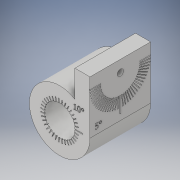
# Autodesk Inventor part: cam_holder_end_part
Saved by Autodesk Inventor 2019 (Build 230136000, 136)
## iProperties
Created: 2024-08-06
Part Number: cam_holder_end_part
Material: Generisch
Document SubType Name: Modeling
Designer: nic
Density: 1 g/cm^3
Appearance: Vorgabe
Author: nic
Autodesk Inventor part; units mm, degrees
ref_plane "YZ Plane" through (0, 0, 0) normal (1, 0, 0) x (0, 1, 0)
ref_plane "XY Plane" through (0, 0, 0) normal (0, 0, 1) x (1, 0, 0)
sketch "Skizze1" plane through (0, 0, 0) normal (0, 0, 1) x (1, 0, 0)
  circle A0 centre (0, 0) radius 10.05
  circle A1 centre (0, 0) radius 20
  line L0 (20, 0) -> (10.05, 0)
  line L1 (10.05, 0) -> (10.05, 35)
  line L2 (10.05, 35) -> (20, 35)
  line L3 (20, 35) -> (20, 0)
  dimension "d1" = 40
  dimension "d0" = 20.1
  dimension "d2" = 35
  constraints: 8 end point, 2 coincident, 2 parallel, 1 centre point, 1 horizontal, 1 horizontal alignment, 1 perpendicular, 2 other
  measures "d0" diameter of A0
  measures "d2" distance of L0.end L1.end
extrude "Extrusion1" add sketch "Skizze1" along normal blind 40
sketch "Skizze2" plane through (0, 0, 40) normal (0, 0, 1) x (1, 0, 0)
  line L0 (7.55, 0.25) -> (12.55, 0.25)
  line L1 (12.55, 0.25) -> (12.55, -0.25)
  line L2 (12.55, -0.25) -> (7.55, -0.25)
  line L3 (7.55, -0.25) -> (7.55, 0.25)
  circle A0 centre (0, 0) radius 10.05 projected
  line L4 (7.55, 0.25) -> (12.55, -0.25) construction
  line L5 (12.55, 0.25) -> (7.55, -0.25) construction
  line L6 (7.384, 1.5941) -> (12.3037, 2.4869)
  line L7 (12.3037, 2.4869) -> (12.393, 1.9949)
  line L8 (12.393, 1.9949) -> (7.4733, 1.1021)
  line L9 (7.4733, 1.1021) -> (7.384, 1.5941)
  line L10 (7.384, 1.5941) -> (12.393, 1.9949) construction
  line L11 (12.3037, 2.4869) -> (7.4733, 1.1021) construction
  line L12 (6.9807, 2.8869) -> (11.6619, 4.6438)
  line L13 (11.6619, 4.6438) -> (11.8376, 4.1757)
  line L14 (11.8376, 4.1757) -> (7.1564, 2.4188)
  line L15 (7.1564, 2.4188) -> (6.9807, 2.8869)
  line L16 (6.9807, 2.8869) -> (11.8376, 4.1757) construction
  line L17 (11.6619, 4.6438) -> (7.1564, 2.4188) construction
  line L18 (6.3531, 4.087) -> (10.6453, 6.6515)
  line L19 (10.6453, 6.6515) -> (10.9018, 6.2223)
  line L20 (10.9018, 6.2223) -> (6.6095, 3.6578)
  line L21 (6.6095, 3.6578) -> (6.3531, 4.087)
  line L22 (6.3531, 4.087) -> (10.9018, 6.2223) construction
  line L23 (10.6453, 6.6515) -> (6.6095, 3.6578) construction
  line L24 (5.5212, 5.1557) -> (9.2866, 8.4454)
  line L25 (9.2866, 8.4454) -> (9.6155, 8.0689)
  line L26 (9.6155, 8.0689) -> (5.8502, 4.7792)
  line L27 (5.8502, 4.7792) -> (5.5212, 5.1557)
  line L28 (5.5212, 5.1557) -> (9.6155, 8.0689) construction
  line L29 (9.2866, 8.4454) -> (5.8502, 4.7792) construction
  line L30 (4.5119, 6.0587) -> (7.6293, 9.9679)
  line L31 (7.6293, 9.9679) -> (8.0203, 9.6561)
  line L32 (8.0203, 9.6561) -> (4.9028, 5.747)
  line L33 (4.9028, 5.747) -> (4.5119, 6.0587)
  line L34 (4.5119, 6.0587) -> (8.0203, 9.6561) construction
  line L35 (7.6293, 9.9679) -> (4.9028, 5.747) construction
  line L36 (3.3576, 6.767) -> (5.7269, 11.1699)
  line L37 (5.7269, 11.1699) -> (6.1672, 10.933)
  line L38 (6.1672, 10.933) -> (3.7979, 6.53)
  line L39 (3.7979, 6.53) -> (3.3576, 6.767)
  line L40 (3.3576, 6.767) -> (6.1672, 10.933) construction
  line L41 (5.7269, 11.1699) -> (3.7979, 6.53) construction
  line L42 (2.0953, 7.2577) -> (3.6404, 12.013)
  line L43 (3.6404, 12.013) -> (4.1159, 11.8585)
  line L44 (4.1159, 11.8585) -> (2.5708, 7.1032)
  line L45 (2.5708, 7.1032) -> (2.0953, 7.2577)
  line L46 (2.0953, 7.2577) -> (4.1159, 11.8585) construction
  line L47 (3.6404, 12.013) -> (2.5708, 7.1032) construction
  line L48 (0.7657, 7.5152) -> (1.4369, 12.47)
  line L49 (1.4369, 12.47) -> (1.9324, 12.4029)
  line L50 (1.9324, 12.4029) -> (1.2612, 7.4481)
  line L51 (1.2612, 7.4481) -> (0.7657, 7.5152)
  line L52 (0.7657, 7.5152) -> (1.9324, 12.4029) construction
  line L53 (1.4369, 12.47) -> (1.2612, 7.4481) construction
  line L54 (-0.5885, 7.5312) -> (-0.8128, 12.5261)
  line L55 (-0.8128, 12.5261) -> (-0.3133, 12.5486)
  line L56 (-0.3133, 12.5486) -> (-0.089, 7.5536)
  line L57 (-0.089, 7.5536) -> (-0.5885, 7.5312)
  line L58 (-0.5885, 7.5312) -> (-0.3133, 12.5486) construction
  line L59 (-0.8128, 12.5261) -> (-0.089, 7.5536) construction
  line L60 (-1.9238, 7.3051) -> (-3.0364, 12.1797)
  line L61 (-3.0364, 12.1797) -> (-2.5489, 12.291)
  line L62 (-2.5489, 12.291) -> (-1.4363, 7.4163)
  line L63 (-1.4363, 7.4163) -> (-1.9238, 7.3051)
  line L64 (-1.9238, 7.3051) -> (-2.5489, 12.291) construction
  line L65 (-3.0364, 12.1797) -> (-1.4363, 7.4163) construction
  line L66 (-3.1972, 6.8442) -> (-5.1623, 11.4418)
  line L67 (-5.1623, 11.4418) -> (-4.7026, 11.6383)
  line L68 (-4.7026, 11.6383) -> (-2.7375, 7.0407)
  line L69 (-2.7375, 7.0407) -> (-3.1972, 6.8442)
  line L70 (-3.1972, 6.8442) -> (-4.7026, 11.6383) construction
  line L71 (-5.1623, 11.4418) -> (-2.7375, 7.0407) construction
  line L72 (-4.3679, 6.1633) -> (-7.1224, 10.3362)
  line L73 (-7.1224, 10.3362) -> (-6.7051, 10.6116)
  line L74 (-6.7051, 10.6116) -> (-3.9506, 6.4388)
  line L75 (-3.9506, 6.4388) -> (-4.3679, 6.1633)
  line L76 (-4.3679, 6.1633) -> (-6.7051, 10.6116) construction
  line L77 (-7.1224, 10.3362) -> (-3.9506, 6.4388) construction
  line L78 (-5.3982, 5.2843) -> (-8.8535, 8.8983)
  line L79 (-8.8535, 8.8983) -> (-8.4921, 9.2438)
  line L80 (-8.4921, 9.2438) -> (-5.0368, 5.6299)
  line L81 (-5.0368, 5.6299) -> (-5.3982, 5.2843)
  line L82 (-5.3982, 5.2843) -> (-8.4921, 9.2438) construction
  line L83 (-8.8535, 8.8983) -> (-5.0368, 5.6299) construction
  line L84 (-6.255, 4.2355) -> (-10.3001, 7.1745)
  line L85 (-10.3001, 7.1745) -> (-10.0062, 7.579)
  line L86 (-10.0062, 7.579) -> (-5.9611, 4.64)
  line L87 (-5.9611, 4.64) -> (-6.255, 4.2355)
  line L88 (-6.255, 4.2355) -> (-10.0062, 7.579) construction
  line L89 (-10.3001, 7.1745) -> (-5.9611, 4.64) construction
  line L90 (-6.9108, 3.0506) -> (-11.4156, 5.22)
  line L91 (-11.4156, 5.22) -> (-11.1987, 5.6705)
  line L92 (-11.1987, 5.6705) -> (-6.6938, 3.5011)
  line L93 (-6.6938, 3.5011) -> (-6.9108, 3.0506)
  line L94 (-6.9108, 3.0506) -> (-11.1987, 5.6705) construction
  line L95 (-11.4156, 5.22) -> (-6.6938, 3.5011) construction
  line L96 (-7.3444, 1.7676) -> (-12.1642, 3.0978)
  line L97 (-12.1642, 3.0978) -> (-12.0312, 3.5798)
  line L98 (-12.0312, 3.5798) -> (-7.2114, 2.2496)
  line L99 (-7.2114, 2.2496) -> (-7.3444, 1.7676)
  line L100 (-7.3444, 1.7676) -> (-12.0312, 3.5798) construction
  line L101 (-12.1642, 3.0978) -> (-7.2114, 2.2496) construction
  line L102 (-7.542, 0.4278) -> (-12.5219, 0.876)
  line L103 (-12.5219, 0.876) -> (-12.4771, 1.374)
  line L104 (-12.4771, 1.374) -> (-7.4972, 0.9258)
  line L105 (-7.4972, 0.9258) -> (-7.542, 0.4278)
  line L106 (-7.542, 0.4278) -> (-12.4771, 1.374) construction
  line L107 (-12.5219, 0.876) -> (-7.4972, 0.9258) construction
  line L108 (-7.4972, -0.9258) -> (-12.4771, -1.374)
  line L109 (-12.4771, -1.374) -> (-12.5219, -0.876)
  line L110 (-12.5219, -0.876) -> (-7.542, -0.4278)
  line L111 (-7.542, -0.4278) -> (-7.4972, -0.9258)
  line L112 (-7.4972, -0.9258) -> (-12.5219, -0.876) construction
  line L113 (-12.4771, -1.374) -> (-7.542, -0.4278) construction
  line L114 (-7.2114, -2.2496) -> (-12.0312, -3.5798)
  line L115 (-12.0312, -3.5798) -> (-12.1642, -3.0978)
  line L116 (-12.1642, -3.0978) -> (-7.3444, -1.7676)
  line L117 (-7.3444, -1.7676) -> (-7.2114, -2.2496)
  line L118 (-7.2114, -2.2496) -> (-12.1642, -3.0978) construction
  line L119 (-12.0312, -3.5798) -> (-7.3444, -1.7676) construction
  line L120 (-6.6938, -3.5011) -> (-11.1987, -5.6705)
  line L121 (-11.1987, -5.6705) -> (-11.4156, -5.22)
  line L122 (-11.4156, -5.22) -> (-6.9108, -3.0506)
  line L123 (-6.9108, -3.0506) -> (-6.6938, -3.5011)
  line L124 (-6.6938, -3.5011) -> (-11.4156, -5.22) construction
  line L125 (-11.1987, -5.6705) -> (-6.9108, -3.0506) construction
  line L126 (-5.9611, -4.64) -> (-10.0062, -7.579)
  line L127 (-10.0062, -7.579) -> (-10.3001, -7.1745)
  line L128 (-10.3001, -7.1745) -> (-6.255, -4.2355)
  line L129 (-6.255, -4.2355) -> (-5.9611, -4.64)
  line L130 (-5.9611, -4.64) -> (-10.3001, -7.1745) construction
  line L131 (-10.0062, -7.579) -> (-6.255, -4.2355) construction
  line L132 (-5.0368, -5.6299) -> (-8.4921, -9.2438)
  line L133 (-8.4921, -9.2438) -> (-8.8535, -8.8983)
  line L134 (-8.8535, -8.8983) -> (-5.3982, -5.2843)
  line L135 (-5.3982, -5.2843) -> (-5.0368, -5.6299)
  line L136 (-5.0368, -5.6299) -> (-8.8535, -8.8983) construction
  line L137 (-8.4921, -9.2438) -> (-5.3982, -5.2843) construction
  line L138 (-3.9506, -6.4388) -> (-6.7051, -10.6116)
  line L139 (-6.7051, -10.6116) -> (-7.1224, -10.3362)
  line L140 (-7.1224, -10.3362) -> (-4.3679, -6.1633)
  line L141 (-4.3679, -6.1633) -> (-3.9506, -6.4388)
  line L142 (-3.9506, -6.4388) -> (-7.1224, -10.3362) construction
  line L143 (-6.7051, -10.6116) -> (-4.3679, -6.1633) construction
  line L144 (-2.7375, -7.0407) -> (-4.7026, -11.6383)
  line L145 (-4.7026, -11.6383) -> (-5.1623, -11.4418)
  line L146 (-5.1623, -11.4418) -> (-3.1972, -6.8442)
  line L147 (-3.1972, -6.8442) -> (-2.7375, -7.0407)
  line L148 (-2.7375, -7.0407) -> (-5.1623, -11.4418) construction
  line L149 (-4.7026, -11.6383) -> (-3.1972, -6.8442) construction
  line L150 (-1.4363, -7.4163) -> (-2.5489, -12.291)
  line L151 (-2.5489, -12.291) -> (-3.0364, -12.1797)
  line L152 (-3.0364, -12.1797) -> (-1.9238, -7.3051)
  line L153 (-1.9238, -7.3051) -> (-1.4363, -7.4163)
  line L154 (-1.4363, -7.4163) -> (-3.0364, -12.1797) construction
  line L155 (-2.5489, -12.291) -> (-1.9238, -7.3051) construction
  line L156 (-0.089, -7.5536) -> (-0.3133, -12.5486)
  line L157 (-0.3133, -12.5486) -> (-0.8128, -12.5261)
  line L158 (-0.8128, -12.5261) -> (-0.5885, -7.5312)
  line L159 (-0.5885, -7.5312) -> (-0.089, -7.5536)
  line L160 (-0.089, -7.5536) -> (-0.8128, -12.5261) construction
  line L161 (-0.3133, -12.5486) -> (-0.5885, -7.5312) construction
  line L162 (1.2612, -7.4481) -> (1.9324, -12.4029)
  line L163 (1.9324, -12.4029) -> (1.4369, -12.47)
  line L164 (1.4369, -12.47) -> (0.7657, -7.5152)
  line L165 (0.7657, -7.5152) -> (1.2612, -7.4481)
  line L166 (1.2612, -7.4481) -> (1.4369, -12.47) construction
  line L167 (1.9324, -12.4029) -> (0.7657, -7.5152) construction
  line L168 (2.5708, -7.1032) -> (4.1159, -11.8585)
  line L169 (4.1159, -11.8585) -> (3.6404, -12.013)
  line L170 (3.6404, -12.013) -> (2.0953, -7.2577)
  line L171 (2.0953, -7.2577) -> (2.5708, -7.1032)
  line L172 (2.5708, -7.1032) -> (3.6404, -12.013) construction
  line L173 (4.1159, -11.8585) -> (2.0953, -7.2577) construction
  line L174 (3.7979, -6.53) -> (6.1672, -10.933)
  line L175 (6.1672, -10.933) -> (5.7269, -11.1699)
  line L176 (5.7269, -11.1699) -> (3.3576, -6.767)
  line L177 (3.3576, -6.767) -> (3.7979, -6.53)
  line L178 (3.7979, -6.53) -> (5.7269, -11.1699) construction
  line L179 (6.1672, -10.933) -> (3.3576, -6.767) construction
  line L180 (4.9028, -5.747) -> (8.0203, -9.6561)
  line L181 (8.0203, -9.6561) -> (7.6293, -9.9679)
  line L182 (7.6293, -9.9679) -> (4.5119, -6.0587)
  line L183 (4.5119, -6.0587) -> (4.9028, -5.747)
  line L184 (4.9028, -5.747) -> (7.6293, -9.9679) construction
  line L185 (8.0203, -9.6561) -> (4.5119, -6.0587) construction
  line L186 (5.8502, -4.7792) -> (9.6155, -8.0689)
  line L187 (9.6155, -8.0689) -> (9.2866, -8.4454)
  line L188 (9.2866, -8.4454) -> (5.5212, -5.1557)
  line L189 (5.5212, -5.1557) -> (5.8502, -4.7792)
  line L190 (5.8502, -4.7792) -> (9.2866, -8.4454) construction
  line L191 (9.6155, -8.0689) -> (5.5212, -5.1557) construction
  line L192 (6.6095, -3.6578) -> (10.9018, -6.2223)
  line L193 (10.9018, -6.2223) -> (10.6453, -6.6515)
  line L194 (10.6453, -6.6515) -> (6.3531, -4.087)
  line L195 (6.3531, -4.087) -> (6.6095, -3.6578)
  line L196 (6.6095, -3.6578) -> (10.6453, -6.6515) construction
  line L197 (10.9018, -6.2223) -> (6.3531, -4.087) construction
  line L198 (7.1564, -2.4188) -> (11.8376, -4.1757)
  line L199 (11.8376, -4.1757) -> (11.6619, -4.6438)
  line L200 (11.6619, -4.6438) -> (6.9807, -2.8869)
  line L201 (6.9807, -2.8869) -> (7.1564, -2.4188)
  line L202 (7.1564, -2.4188) -> (11.6619, -4.6438) construction
  line L203 (11.8376, -4.1757) -> (6.9807, -2.8869) construction
  line L204 (7.4733, -1.1021) -> (12.393, -1.9949)
  line L205 (12.393, -1.9949) -> (12.3037, -2.4869)
  line L206 (12.3037, -2.4869) -> (7.384, -1.5941)
  line L207 (7.384, -1.5941) -> (7.4733, -1.1021)
  line L208 (7.4733, -1.1021) -> (12.3037, -2.4869) construction
  line L209 (12.393, -1.9949) -> (7.384, -1.5941) construction
  line L210 (4.9213, 0.25) -> (15.1787, 0.25)
  line L211 (15.1787, 0.25) -> (15.1787, -0.25)
  line L212 (15.1787, -0.25) -> (4.9213, -0.25)
  line L213 (4.9213, -0.25) -> (4.9213, 0.25)
  line L214 (4.9213, 0.25) -> (15.1787, -0.25) construction
  line L215 (15.1787, 0.25) -> (4.9213, -0.25) construction
  point P0 (10.05, 0)
  point P1 (9.8885, 1.7945)
  point P2 (9.4092, 3.5313)
  point P3 (8.6274, 5.1546)
  point P4 (7.5684, 6.6123)
  point P5 (6.2661, 7.8574)
  point P6 (4.7624, 8.85)
  point P7 (3.1056, 9.5581)
  point P8 (1.349, 9.959)
  point P9 (-0.4509, 10.0399)
  point P10 (-2.2363, 9.798)
  point P11 (-3.9499, 9.2413)
  point P12 (-5.5365, 8.3875)
  point P13 (-6.9452, 7.2641)
  point P14 (-8.1306, 5.9072)
  point P15 (-9.0547, 4.3605)
  point P16 (-9.6878, 2.6737)
  point P17 (-10.0095, 0.9009)
  point P18 (-10.0095, -0.9009)
  point P19 (-9.6878, -2.6737)
  point P20 (-9.0547, -4.3605)
  point P21 (-8.1306, -5.9072)
  point P22 (-6.9452, -7.2641)
  point P23 (-5.5365, -8.3875)
  point P24 (-3.9499, -9.2413)
  point P25 (-2.2363, -9.798)
  point P26 (-0.4509, -10.0399)
  point P27 (1.349, -9.959)
  point P28 (3.1056, -9.5581)
  point P29 (4.7624, -8.85)
  point P30 (6.2661, -7.8574)
  point P31 (7.5684, -6.6123)
  point P32 (8.6274, -5.1546)
  point P33 (9.4092, -3.5313)
  point P34 (9.8885, -1.7945)
  dimension "d5" = 5
  dimension "d6" = 0.5
  dimension "d9" = 360
  constraints: 432 end point, 72 midpoint, 4 parallel, 2 horizontal, 2 perpendicular, 1 horizontal alignment, 387 other
  measures "d5" distance of L1.end L2.end
  measures "d6" distance of L0.end L1.end
extrude "Extrusion2" cut sketch "Skizze2" against normal blind 0.5 contours L0 A0 L2 L3 | L3 L212 L213 L210 | L0 L1 L2 A0 | L210 L211 L212 L1 | L8 L9 L6 A0 | A0 L6 L7 L8 | L204 L205 L206 A0 | A0 L206 L207 L204 | L14 L15 L12 A0 | A0 L12 L13 L14 | L198 L199 L200 A0 | A0 L200 L201 L198 | L20 L21 L18 A0 | A0 L18 L19 L20 | L192 L193 L194 A0 | A0 L194 L195 L192 | L26 L27 L24 A0 | A0 L24 L25 L26 | L186 L187 L188 A0 | A0 L188 L189 L186 | L32 L33 L30 A0 | A0 L30 L31 L32 | L180 L181 L182 A0 | A0 L182 L183 L180 | L38 L39 L36 A0 | A0 L36 L37 L38 | L174 L175 L176 A0 | A0 L176 L177 L174 | L44 L45 L42 A0 | A0 L42 L43 L44 | L168 L169 L170 A0 | A0 L170 L171 L168 | L50 L51 L48 A0 | A0 L48 L49 L50 | L162 L163 L164 A0 | A0 L164 L165 L162 | L56 L57 L54 A0 | A0 L54 L55 L56 | L156 L157 L158 A0 | A0 L158 L159 L156 | L62 L63 L60 A0 | A0 L60 L61 L62 | L150 L151 L152 A0 | A0 L152 L153 L150 | L68 L69 L66 A0 | A0 L66 L67 L68 | L144 L145 L146 A0 | A0 L146 L147 L144 | L74 L75 L72 A0 | A0 L72 L73 L74 | L138 L139 L140 A0 | A0 L140 L141 L138 | L80 L81 L78 A0 | A0 L78 L79 L80 | L132 L133 L134 A0 | A0 L134 L135 L132 | L86 L87 L84 A0 | A0 L84 L85 L86 | L126 L127 L128 A0 | A0 L128 L129 L126 | L92 L93 L90 A0 | A0 L90 L91 L92 | L120 L121 L122 A0 | A0 L122 L123 L120 | L98 L99 L96 A0 | A0 L96 L97 L98 | L114 L115 L116 A0 | A0 L116 L117 L114 | L104 L105 L102 A0 | A0 L102 L103 L104 | L108 L109 L110 A0 | A0 L110 L111 L108
sketch "Skizze3" plane through (10.05, 17.2915, 0) normal (-1, 0, 0) x (0, 0, 1)
  line L0 (0, 0) -> (40, 0) construction
  line L1 (40, 17.7085) -> (40, 0) construction
  line L2 (0, 17.7085) -> (40, 17.7085) construction
  line L3 (0, 0) -> (0, 17.7085) construction
  line L4 (0, 17.7085) -> (40, 17.7085) projected
  line L5 (20, 17.7085) -> (20, 7.753)
  line L6 (40, 17.7085) -> (40, 0) projected
  line L7 (40, 10.1178) -> (0, 10.1178)
  point P0 (0, -17.2915)
  point P1 (20, 10.1178)
  constraints: 4 end point, 2 midpoint, 2 point on line, 1 perpendicular, 1 vertical
hole "Bohrung1" at (10.05, 27.4094, 20) direction (1, 0, 0) diameter 4.1 depth 20 tip angle 118 counterbore diameter 8 counterbore depth 3 clearance for "Zylinderschraube mit Schlitz DIN 84" size "M4" standard "DIN"
ref_plane "Arbeitsebene1" through (0, -20, 0) normal (0, 1, 0) x (-1, 0, 0)
sketch "Skizze4" plane through (0, -20, 0) normal (0, 1, 0) x (-1, 0, 0)
  line L0 (-10.05, 0) -> (-10.05, 40) construction
  line L1 (-20, 0) -> (-10.05, 0) construction
  line L2 (-20, 0) -> (-20, 40) construction
  line L3 (-10.05, 40) -> (-20, 40) construction
  line L4 (0, 40) -> (0, 0)
  point P0 (0, 20)
  constraints: 2 end point, 1 midpoint, 1 vertical
hole "Bohrung2" at (0, -20, 20) direction (0, 1, 0) diameter 4.1 depth 12 tip angle 118 counterbore diameter 5 counterbore depth 2
sketch "Skizze6" plane through (10.05, 17.2915, 0) normal (-1, 0, 0) x (0, 0, 1)
  circle A0 centre (20, 10.1178) radius 2.05 projected
  circle A1 centre (20, 10.1178) radius 4
  circle A2 centre (20, 10.1178) radius 2.05
  point P0 (0, -17.2915)
  dimension "d37" = 4.1
  constraints: 2 centre point, 2 coincident
  measures "d37" diameter of A2
extrude "Extrusion4" add sketch "Skizze6" against normal up to surface (3 mm away)
sketch "Skizze7" plane through (20, 0, 0) normal (1, 0, 0) x (0, 0, -1)
  circle A0 centre (-20, 27.4094) radius 2.05 construction
  circle A1 centre (-20, 27.4094) radius 13 construction
  circle A2 centre (-20, 27.4094) radius 20 construction
  line L0 (0, 17.2915) -> (-40, 17.2915) projected
  line L1 (-20.5, 17.2915) -> (-20, 17.2915)
  line L2 (-20, 14.4094) -> (-20.25, 14.4094)
  line L3 (-20.25, 7.4109) -> (-19.75, 7.4109)
  line L4 (-19.75, 21.4078) -> (-20.25, 7.4109) construction
  line L5 (-20.25, 21.4078) -> (-19.75, 7.4109) construction
  line L6 (-19.75, 14.4094) -> (-20.25, 14.4094)
  line L7 (-20.25, 14.4118) -> (-20.25, 7.4109)
  line L8 (-19.75, 7.4109) -> (-19.75, 14.4118)
  line L9 (-18.867, 14.4588) -> (-19.116, 14.437)
  line L10 (-18.5061, 7.4652) -> (-18.008, 7.5088)
  line L11 (-18.6179, 14.4806) -> (-19.116, 14.437)
  line L12 (-19.1162, 14.4394) -> (-18.5061, 7.4652)
  line L13 (-18.008, 7.5088) -> (-18.6181, 14.483)
  line L14 (-17.7426, 14.6069) -> (-17.9888, 14.5634)
  line L15 (-16.7735, 7.6713) -> (-16.2811, 7.7582)
  line L16 (-17.4964, 14.6503) -> (-17.9888, 14.5634)
  line L17 (-17.9892, 14.5658) -> (-16.7735, 7.6713)
  line L18 (-16.2811, 7.7582) -> (-17.4968, 14.6526)
  line L19 (-16.6354, 14.8523) -> (-16.8768, 14.7876)
  line L20 (-15.0655, 8.0276) -> (-14.5825, 8.1571)
  line L21 (-16.3939, 14.917) -> (-16.8768, 14.7876)
  line L22 (-16.8775, 14.7899) -> (-15.0655, 8.0276)
  line L23 (-14.5825, 8.1571) -> (-16.3945, 14.9194)
  line L24 (-15.5537, 15.1934) -> (-15.7887, 15.1079)
  line L25 (-13.3951, 8.5315) -> (-12.9252, 8.7025)
  line L26 (-15.3188, 15.2789) -> (-15.7887, 15.1079)
  line L27 (-15.7895, 15.1101) -> (-13.3951, 8.5315)
  line L28 (-12.9252, 8.7025) -> (-15.3196, 15.2811)
  line L29 (-14.506, 15.6274) -> (-14.7325, 15.5217)
  line L30 (-11.7749, 9.179) -> (-11.3217, 9.3903)
  line L31 (-14.2794, 15.733) -> (-14.7325, 15.5217)
  line L32 (-14.7336, 15.5239) -> (-11.7749, 9.179)
  line L33 (-11.3217, 9.3903) -> (-14.2804, 15.7352)
  line L34 (-13.5, 16.151) -> (-13.7165, 16.026)
  line L35 (-10.2173, 9.9652) -> (-9.7843, 10.2152)
  line L36 (-13.2835, 16.276) -> (-13.7165, 16.026)
  line L37 (-13.7177, 16.0281) -> (-10.2173, 9.9652)
  line L38 (-9.7843, 10.2152) -> (-13.2847, 16.2781)
  line L39 (-12.5435, 16.7604) -> (-12.7483, 16.617)
  line L40 (-8.7342, 10.8842) -> (-8.3246, 11.171)
  line L41 (-12.3387, 16.9038) -> (-12.7483, 16.617)
  line L42 (-12.7497, 16.619) -> (-8.7342, 10.8842)
  line L43 (-8.3246, 11.171) -> (-12.3401, 16.9057)
  line L44 (-11.6438, 17.4508) -> (-11.8353, 17.2901)
  line L45 (-7.3368, 11.929) -> (-6.9537, 12.2504)
  line L46 (-11.4522, 17.6115) -> (-11.8353, 17.2901)
  line L47 (-11.8368, 17.2919) -> (-7.3368, 11.929)
  line L48 (-6.9537, 12.2504) -> (-11.4538, 17.6133)
  line L49 (-10.8076, 18.217) -> (-10.9844, 18.0402)
  line L50 (-6.0357, 13.0916) -> (-5.6822, 13.4451)
  line L51 (-10.6308, 18.3937) -> (-10.9844, 18.0402)
  line L52 (-10.9861, 18.0419) -> (-6.0357, 13.0916)
  line L53 (-5.6822, 13.4451) -> (-10.6325, 18.3954)
  line L54 (-10.0414, 19.0531) -> (-10.2021, 18.8616)
  line L55 (-4.841, 14.3631) -> (-4.5196, 14.7461)
  line L56 (-9.8807, 19.2446) -> (-10.2021, 18.8616)
  line L57 (-10.204, 18.8632) -> (-4.841, 14.3631)
  line L58 (-4.5196, 14.7461) -> (-9.8826, 19.2462)
  line L59 (-9.351, 19.9529) -> (-9.4944, 19.7481)
  line L60 (-3.7616, 15.7339) -> (-3.4748, 16.1435)
  line L61 (-9.2076, 20.1577) -> (-9.4944, 19.7481)
  line L62 (-9.4964, 19.7495) -> (-3.7616, 15.7339)
  line L63 (-3.4748, 16.1435) -> (-9.2096, 20.159)
  line L64 (-8.7417, 20.9094) -> (-8.8667, 20.6929)
  line L65 (-2.8058, 17.1936) -> (-2.5558, 17.6266)
  line L66 (-8.6167, 21.1259) -> (-8.8667, 20.6929)
  line L67 (-8.8688, 20.6941) -> (-2.8058, 17.1936)
  line L68 (-2.5558, 17.6266) -> (-8.6188, 21.1271)
  line L69 (-8.218, 21.9153) -> (-8.3237, 21.6887)
  line L70 (-1.9809, 18.7311) -> (-1.7696, 19.1842)
  line L71 (-8.1123, 22.1419) -> (-8.3237, 21.6887)
  line L72 (-8.3258, 21.6898) -> (-1.9809, 18.7311)
  line L73 (-1.7696, 19.1842) -> (-8.1145, 22.1429)
  line L74 (-7.784, 22.9631) -> (-7.8695, 22.7282)
  line L75 (-1.2931, 20.3346) -> (-1.1221, 20.8044)
  line L76 (-7.6985, 23.198) -> (-7.8695, 22.7282)
  line L77 (-7.8718, 22.729) -> (-1.2931, 20.3346)
  line L78 (-1.1221, 20.8044) -> (-7.7007, 23.1988)
  line L79 (-7.443, 24.0447) -> (-7.5077, 23.8032)
  line L80 (-0.7477, 21.9919) -> (-0.6183, 22.4749)
  line L81 (-7.3783, 24.2862) -> (-7.5077, 23.8032)
  line L82 (-7.51, 23.8039) -> (-0.7477, 21.9919)
  line L83 (-0.6183, 22.4749) -> (-7.3806, 24.2868)
  line L84 (-7.1975, 25.1519) -> (-7.2409, 24.9057)
  line L85 (-0.3488, 23.6905) -> (-0.262, 24.1829)
  line L86 (-7.1541, 25.3981) -> (-7.2409, 24.9057)
  line L87 (-7.2433, 24.9061) -> (-0.3488, 23.6905)
  line L88 (-0.262, 24.1829) -> (-7.1565, 25.3986)
  line L89 (-7.0495, 26.2763) -> (-7.0713, 26.0273)
  line L90 (-0.0995, 25.4173) -> (-0.0559, 25.9154)
  line L91 (-7.0277, 26.5254) -> (-7.0713, 26.0273)
  line L92 (-7.0737, 26.0275) -> (-0.0995, 25.4173)
  line L93 (-0.0559, 25.9154) -> (-7.0301, 26.5256)
  line L94 (-7, 27.4094) -> (-7, 27.1594)
  line L95 (-0.0016, 27.1594) -> (-0.0016, 27.6594)
  line L96 (-7, 27.6594) -> (-7, 27.1594)
  line L97 (-7.0024, 27.1594) -> (-0.0016, 27.1594)
  line L98 (-0.0016, 27.6594) -> (-7.0024, 27.6594)
  line L99 (-7.0495, 28.5424) -> (-7.0277, 28.2933)
  line L100 (-0.0559, 28.9033) -> (-0.0995, 29.4014)
  line L101 (-7.0713, 28.7914) -> (-7.0277, 28.2933)
  line L102 (-7.0301, 28.2931) -> (-0.0559, 28.9033)
  line L103 (-0.0995, 29.4014) -> (-7.0737, 28.7912)
  line L104 (-7.1975, 29.6668) -> (-7.1541, 29.4206)
  line L105 (-0.262, 30.6358) -> (-0.3488, 31.1283)
  line L106 (-7.2409, 29.913) -> (-7.1541, 29.4206)
  line L107 (-7.1565, 29.4202) -> (-0.262, 30.6358)
  line L108 (-0.3488, 31.1283) -> (-7.2433, 29.9126)
  line L109 (-7.443, 30.774) -> (-7.3783, 30.5325)
  line L110 (-0.6183, 32.3439) -> (-0.7477, 32.8268)
  line L111 (-7.5077, 31.0155) -> (-7.3783, 30.5325)
  line L112 (-7.3806, 30.5319) -> (-0.6183, 32.3439)
  line L113 (-0.7477, 32.8268) -> (-7.51, 31.0149)
  line L114 (-7.784, 31.8556) -> (-7.6985, 31.6207)
  line L115 (-1.1221, 34.0143) -> (-1.2931, 34.4842)
  line L116 (-7.8695, 32.0905) -> (-7.6985, 31.6207)
  line L117 (-7.7007, 31.6199) -> (-1.1221, 34.0143)
  line L118 (-1.2931, 34.4842) -> (-7.8718, 32.0897)
  line L119 (-8.218, 32.9034) -> (-8.1123, 32.6768)
  line L120 (-1.7696, 35.6345) -> (-1.9809, 36.0876)
  line L121 (-8.3237, 33.13) -> (-8.1123, 32.6768)
  line L122 (-8.1145, 32.6758) -> (-1.7696, 35.6345)
  line L123 (-1.9809, 36.0876) -> (-8.3258, 33.129)
  line L124 (-8.7417, 33.9094) -> (-8.6167, 33.6929)
  line L125 (-2.5558, 37.1921) -> (-2.8058, 37.6251)
  line L126 (-8.8667, 34.1259) -> (-8.6167, 33.6929)
  line L127 (-8.6188, 33.6917) -> (-2.5558, 37.1921)
  line L128 (-2.8058, 37.6251) -> (-8.8688, 34.1247)
  line L129 (-9.351, 34.8659) -> (-9.2076, 34.6611)
  line L130 (-3.4748, 38.6752) -> (-3.7616, 39.0848)
  line L131 (-9.4944, 35.0706) -> (-9.2076, 34.6611)
  line L132 (-9.2096, 34.6597) -> (-3.4748, 38.6752)
  line L133 (-3.7616, 39.0848) -> (-9.4964, 35.0693)
  line L134 (-10.0414, 35.7656) -> (-9.8807, 35.5741)
  line L135 (-4.5196, 40.0726) -> (-4.841, 40.4556)
  line L136 (-10.2021, 35.9571) -> (-9.8807, 35.5741)
  line L137 (-9.8826, 35.5725) -> (-4.5196, 40.0726)
  line L138 (-4.841, 40.4556) -> (-10.204, 35.9556)
  line L139 (-10.8076, 36.6017) -> (-10.6308, 36.425)
  line L140 (-5.6822, 41.3736) -> (-6.0357, 41.7272)
  line L141 (-10.9844, 36.7785) -> (-10.6308, 36.425)
  line L142 (-10.6325, 36.4233) -> (-5.6822, 41.3736)
  line L143 (-6.0357, 41.7272) -> (-10.9861, 36.7768)
  line L144 (-11.6438, 37.3679) -> (-11.4522, 37.2072)
  line L145 (-6.9537, 42.5684) -> (-7.3368, 42.8897)
  line L146 (-11.8353, 37.5286) -> (-11.4522, 37.2072)
  line L147 (-11.4538, 37.2054) -> (-6.9537, 42.5684)
  line L148 (-7.3368, 42.8897) -> (-11.8368, 37.5268)
  line L149 (-12.5435, 38.0583) -> (-12.3387, 37.9149)
  line L150 (-8.3246, 43.6477) -> (-8.7342, 43.9345)
  line L151 (-12.7483, 38.2017) -> (-12.3387, 37.9149)
  line L152 (-12.3401, 37.913) -> (-8.3246, 43.6477)
  line L153 (-8.7342, 43.9345) -> (-12.7497, 38.1998)
  line L154 (-13.5, 38.6677) -> (-13.2835, 38.5427)
  line L155 (-9.7843, 44.6035) -> (-10.2173, 44.8535)
  line L156 (-13.7165, 38.7927) -> (-13.2835, 38.5427)
  line L157 (-13.2847, 38.5406) -> (-9.7843, 44.6035)
  line L158 (-10.2173, 44.8535) -> (-13.7177, 38.7906)
  line L159 (-14.506, 39.1914) -> (-14.2794, 39.0857)
  line L160 (-11.3217, 45.4284) -> (-11.7749, 45.6398)
  line L161 (-14.7325, 39.297) -> (-14.2794, 39.0857)
  line L162 (-14.2804, 39.0835) -> (-11.3217, 45.4284)
  line L163 (-11.7749, 45.6398) -> (-14.7336, 39.2948)
  line L164 (-15.5537, 39.6254) -> (-15.3188, 39.5399)
  line L165 (-12.9252, 46.1162) -> (-13.3951, 46.2872)
  line L166 (-15.7887, 39.7109) -> (-15.3188, 39.5399)
  line L167 (-15.3196, 39.5376) -> (-12.9252, 46.1162)
  line L168 (-13.3951, 46.2872) -> (-15.7895, 39.7086)
  line L169 (-16.6354, 39.9664) -> (-16.3939, 39.9017)
  line L170 (-14.5825, 46.6617) -> (-15.0655, 46.7911)
  line L171 (-16.8768, 40.0311) -> (-16.3939, 39.9017)
  line L172 (-16.3945, 39.8994) -> (-14.5825, 46.6617)
  line L173 (-15.0655, 46.7911) -> (-16.8775, 40.0288)
  line L174 (-17.7426, 40.2119) -> (-17.4964, 40.1684)
  line L175 (-16.2811, 47.0606) -> (-16.7735, 47.1474)
  line L176 (-17.9888, 40.2553) -> (-17.4964, 40.1684)
  line L177 (-17.4968, 40.1661) -> (-16.2811, 47.0606)
  line L178 (-16.7735, 47.1474) -> (-17.9892, 40.2529)
  line L179 (-18.867, 40.3599) -> (-18.6179, 40.3381)
  line L180 (-18.008, 47.3099) -> (-18.5061, 47.3535)
  line L181 (-19.116, 40.3817) -> (-18.6179, 40.3381)
  line L182 (-18.6181, 40.3357) -> (-18.008, 47.3099)
  line L183 (-18.5061, 47.3535) -> (-19.1162, 40.3793)
  line L184 (-20, 40.4094) -> (-19.75, 40.4094)
  line L185 (-19.75, 47.4078) -> (-20.25, 47.4078)
  line L186 (-20.25, 40.4094) -> (-19.75, 40.4094)
  line L187 (-19.75, 40.407) -> (-19.75, 47.4078)
  line L188 (-20.25, 47.4078) -> (-20.25, 40.407)
  line L189 (-21.133, 40.3599) -> (-20.884, 40.3817)
  line L190 (-21.4939, 47.3535) -> (-21.992, 47.3099)
  line L191 (-21.3821, 40.3381) -> (-20.884, 40.3817)
  line L192 (-20.8838, 40.3793) -> (-21.4939, 47.3535)
  line L193 (-21.992, 47.3099) -> (-21.3819, 40.3357)
  line L194 (-22.2574, 40.2119) -> (-22.0112, 40.2553)
  line L195 (-23.2265, 47.1474) -> (-23.7189, 47.0606)
  line L196 (-22.5036, 40.1684) -> (-22.0112, 40.2553)
  line L197 (-22.0108, 40.2529) -> (-23.2265, 47.1474)
  line L198 (-23.7189, 47.0606) -> (-22.5032, 40.1661)
  line L199 (-23.3646, 39.9664) -> (-23.1232, 40.0311)
  line L200 (-24.9345, 46.7911) -> (-25.4175, 46.6617)
  line L201 (-23.6061, 39.9017) -> (-23.1232, 40.0311)
  line L202 (-23.1225, 40.0288) -> (-24.9345, 46.7911)
  line L203 (-25.4175, 46.6617) -> (-23.6055, 39.8994)
  line L204 (-24.4463, 39.6254) -> (-24.2113, 39.7109)
  line L205 (-26.6049, 46.2872) -> (-27.0748, 46.1162)
  line L206 (-24.6812, 39.5399) -> (-24.2113, 39.7109)
  line L207 (-24.2105, 39.7086) -> (-26.6049, 46.2872)
  line L208 (-27.0748, 46.1162) -> (-24.6804, 39.5376)
  line L209 (-25.494, 39.1914) -> (-25.2675, 39.297)
  line L210 (-28.2251, 45.6398) -> (-28.6783, 45.4284)
  line L211 (-25.7206, 39.0857) -> (-25.2675, 39.297)
  line L212 (-25.2664, 39.2948) -> (-28.2251, 45.6398)
  line L213 (-28.6783, 45.4284) -> (-25.7196, 39.0835)
  line L214 (-26.5, 38.6677) -> (-26.2835, 38.7927)
  line L215 (-29.7827, 44.8535) -> (-30.2157, 44.6035)
  line L216 (-26.7165, 38.5427) -> (-26.2835, 38.7927)
  line L217 (-26.2823, 38.7906) -> (-29.7827, 44.8535)
  line L218 (-30.2157, 44.6035) -> (-26.7153, 38.5406)
  line L219 (-27.4565, 38.0583) -> (-27.2517, 38.2017)
  line L220 (-31.2658, 43.9345) -> (-31.6754, 43.6477)
  line L221 (-27.6613, 37.9149) -> (-27.2517, 38.2017)
  line L222 (-27.2503, 38.1998) -> (-31.2658, 43.9345)
  line L223 (-31.6754, 43.6477) -> (-27.6599, 37.913)
  line L224 (-28.3562, 37.3679) -> (-28.1647, 37.5286)
  line L225 (-32.6632, 42.8897) -> (-33.0463, 42.5684)
  line L226 (-28.5478, 37.2072) -> (-28.1647, 37.5286)
  line L227 (-28.1632, 37.5268) -> (-32.6632, 42.8897)
  line L228 (-33.0463, 42.5684) -> (-28.5462, 37.2054)
  line L229 (-29.1924, 36.6017) -> (-29.0156, 36.7785)
  line L230 (-33.9643, 41.7272) -> (-34.3178, 41.3736)
  line L231 (-29.3692, 36.425) -> (-29.0156, 36.7785)
  line L232 (-29.0139, 36.7768) -> (-33.9643, 41.7272)
  line L233 (-34.3178, 41.3736) -> (-29.3675, 36.4233)
  line L234 (-29.9586, 35.7656) -> (-29.7979, 35.9571)
  line L235 (-35.159, 40.4556) -> (-35.4804, 40.0726)
  line L236 (-30.1193, 35.5741) -> (-29.7979, 35.9571)
  line L237 (-29.796, 35.9556) -> (-35.159, 40.4556)
  line L238 (-35.4804, 40.0726) -> (-30.1174, 35.5725)
  line L239 (-30.649, 34.8659) -> (-30.5056, 35.0706)
  line L240 (-36.2384, 39.0848) -> (-36.5252, 38.6752)
  line L241 (-30.7924, 34.6611) -> (-30.5056, 35.0706)
  line L242 (-30.5036, 35.0693) -> (-36.2384, 39.0848)
  line L243 (-36.5252, 38.6752) -> (-30.7904, 34.6597)
  line L244 (-31.2583, 33.9094) -> (-31.1333, 34.1259)
  line L245 (-37.1942, 37.6251) -> (-37.4442, 37.1921)
  line L246 (-31.3833, 33.6929) -> (-31.1333, 34.1259)
  line L247 (-31.1312, 34.1247) -> (-37.1942, 37.6251)
  line L248 (-37.4442, 37.1921) -> (-31.3812, 33.6917)
  line L249 (-31.782, 32.9034) -> (-31.6763, 33.13)
  line L250 (-38.0191, 36.0876) -> (-38.2304, 35.6345)
  line L251 (-31.8877, 32.6768) -> (-31.6763, 33.13)
  line L252 (-31.6742, 33.129) -> (-38.0191, 36.0876)
  line L253 (-38.2304, 35.6345) -> (-31.8855, 32.6758)
  line L254 (-32.216, 31.8556) -> (-32.1305, 32.0905)
  line L255 (-38.7069, 34.4842) -> (-38.8779, 34.0143)
  line L256 (-32.3015, 31.6207) -> (-32.1305, 32.0905)
  line L257 (-32.1282, 32.0897) -> (-38.7069, 34.4842)
  line L258 (-38.8779, 34.0143) -> (-32.2993, 31.6199)
  line L259 (-32.557, 30.774) -> (-32.4923, 31.0155)
  line L260 (-39.2523, 32.8268) -> (-39.3817, 32.3439)
  line L261 (-32.6217, 30.5325) -> (-32.4923, 31.0155)
  line L262 (-32.49, 31.0149) -> (-39.2523, 32.8268)
  line L263 (-39.3817, 32.3439) -> (-32.6194, 30.5319)
  line L264 (-32.8025, 29.6668) -> (-32.7591, 29.913)
  line L265 (-39.6512, 31.1283) -> (-39.738, 30.6358)
  line L266 (-32.8459, 29.4206) -> (-32.7591, 29.913)
  line L267 (-32.7567, 29.9126) -> (-39.6512, 31.1283)
  line L268 (-39.738, 30.6358) -> (-32.8435, 29.4202)
  line L269 (-32.9505, 28.5424) -> (-32.9287, 28.7914)
  line L270 (-39.9005, 29.4014) -> (-39.9441, 28.9033)
  line L271 (-32.9723, 28.2933) -> (-32.9287, 28.7914)
  line L272 (-32.9263, 28.7912) -> (-39.9005, 29.4014)
  line L273 (-39.9441, 28.9033) -> (-32.9699, 28.2931)
  line L274 (-33, 27.4094) -> (-33, 27.6594)
  line L275 (-39.9984, 27.6594) -> (-39.9984, 27.1594)
  line L276 (-33, 27.1594) -> (-33, 27.6594)
  line L277 (-32.9976, 27.6594) -> (-39.9984, 27.6594)
  line L278 (-39.9984, 27.1594) -> (-32.9976, 27.1594)
  line L279 (-32.9505, 26.2763) -> (-32.9723, 26.5254)
  line L280 (-39.9441, 25.9154) -> (-39.9005, 25.4173)
  line L281 (-32.9287, 26.0273) -> (-32.9723, 26.5254)
  line L282 (-32.9699, 26.5256) -> (-39.9441, 25.9154)
  line L283 (-39.9005, 25.4173) -> (-32.9263, 26.0275)
  line L284 (-32.8025, 25.1519) -> (-32.8459, 25.3981)
  line L285 (-39.738, 24.1829) -> (-39.6512, 23.6905)
  line L286 (-32.7591, 24.9057) -> (-32.8459, 25.3981)
  line L287 (-32.8435, 25.3986) -> (-39.738, 24.1829)
  line L288 (-39.6512, 23.6905) -> (-32.7567, 24.9061)
  line L289 (-32.557, 24.0447) -> (-32.6217, 24.2862)
  line L290 (-39.3817, 22.4749) -> (-39.2523, 21.9919)
  line L291 (-32.4923, 23.8032) -> (-32.6217, 24.2862)
  line L292 (-32.6194, 24.2868) -> (-39.3817, 22.4749)
  line L293 (-39.2523, 21.9919) -> (-32.49, 23.8039)
  line L294 (-32.216, 22.9631) -> (-32.3015, 23.198)
  line L295 (-38.8779, 20.8044) -> (-38.7069, 20.3346)
  line L296 (-32.1305, 22.7282) -> (-32.3015, 23.198)
  line L297 (-32.2993, 23.1988) -> (-38.8779, 20.8044)
  line L298 (-38.7069, 20.3346) -> (-32.1282, 22.729)
  line L299 (-31.782, 21.9153) -> (-31.8877, 22.1419)
  line L300 (-38.2304, 19.1842) -> (-38.0191, 18.7311)
  line L301 (-31.6763, 21.6887) -> (-31.8877, 22.1419)
  line L302 (-31.8855, 22.1429) -> (-38.2304, 19.1842)
  line L303 (-38.0191, 18.7311) -> (-31.6742, 21.6898)
  line L304 (-31.2583, 20.9094) -> (-31.3833, 21.1259)
  line L305 (-37.4442, 17.6266) -> (-37.1942, 17.1936)
  line L306 (-31.1333, 20.6929) -> (-31.3833, 21.1259)
  line L307 (-31.3812, 21.1271) -> (-37.4442, 17.6266)
  line L308 (-37.1942, 17.1936) -> (-31.1312, 20.6941)
  line L309 (-30.649, 19.9529) -> (-30.7924, 20.1577)
  line L310 (-36.5252, 16.1435) -> (-36.2384, 15.7339)
  line L311 (-30.5056, 19.7481) -> (-30.7924, 20.1577)
  line L312 (-30.7904, 20.159) -> (-36.5252, 16.1435)
  line L313 (-36.2384, 15.7339) -> (-30.5036, 19.7495)
  line L314 (-29.9586, 19.0531) -> (-30.1193, 19.2446)
  line L315 (-35.4804, 14.7461) -> (-35.159, 14.3631)
  line L316 (-29.7979, 18.8616) -> (-30.1193, 19.2446)
  line L317 (-30.1174, 19.2462) -> (-35.4804, 14.7461)
  line L318 (-35.159, 14.3631) -> (-29.796, 18.8632)
  line L319 (-29.1924, 18.217) -> (-29.3692, 18.3937)
  line L320 (-34.3178, 13.4451) -> (-33.9643, 13.0916)
  line L321 (-29.0156, 18.0402) -> (-29.3692, 18.3937)
  line L322 (-29.3675, 18.3954) -> (-34.3178, 13.4451)
  line L323 (-33.9643, 13.0916) -> (-29.0139, 18.0419)
  line L324 (-28.3562, 17.4508) -> (-28.5478, 17.6115)
  line L325 (-33.0463, 12.2504) -> (-32.6632, 11.929)
  line L326 (-28.1647, 17.2901) -> (-28.5478, 17.6115)
  line L327 (-28.5462, 17.6133) -> (-33.0463, 12.2504)
  line L328 (-32.6632, 11.929) -> (-28.1632, 17.2919)
  line L329 (-27.4565, 16.7604) -> (-27.6613, 16.9038)
  line L330 (-31.6754, 11.171) -> (-31.2658, 10.8842)
  line L331 (-27.2517, 16.617) -> (-27.6613, 16.9038)
  line L332 (-27.6599, 16.9057) -> (-31.6754, 11.171)
  line L333 (-31.2658, 10.8842) -> (-27.2503, 16.619)
  line L334 (-26.5, 16.151) -> (-26.7165, 16.276)
  line L335 (-30.2157, 10.2152) -> (-29.7827, 9.9652)
  line L336 (-26.2835, 16.026) -> (-26.7165, 16.276)
  line L337 (-26.7153, 16.2781) -> (-30.2157, 10.2152)
  line L338 (-29.7827, 9.9652) -> (-26.2823, 16.0281)
  line L339 (-25.494, 15.6274) -> (-25.7206, 15.733)
  line L340 (-28.6783, 9.3903) -> (-28.2251, 9.179)
  line L341 (-25.2675, 15.5217) -> (-25.7206, 15.733)
  line L342 (-25.7196, 15.7352) -> (-28.6783, 9.3903)
  line L343 (-28.2251, 9.179) -> (-25.2664, 15.5239)
  line L344 (-24.4463, 15.1934) -> (-24.6812, 15.2789)
  line L345 (-27.0748, 8.7025) -> (-26.6049, 8.5315)
  line L346 (-24.2113, 15.1079) -> (-24.6812, 15.2789)
  line L347 (-24.6804, 15.2811) -> (-27.0748, 8.7025)
  line L348 (-26.6049, 8.5315) -> (-24.2105, 15.1101)
  line L349 (-23.3646, 14.8523) -> (-23.6061, 14.917)
  line L350 (-25.4175, 8.1571) -> (-24.9345, 8.0276)
  line L351 (-23.1232, 14.7876) -> (-23.6061, 14.917)
  line L352 (-23.6055, 14.9194) -> (-25.4175, 8.1571)
  line L353 (-24.9345, 8.0276) -> (-23.1225, 14.7899)
  line L354 (-22.2574, 14.6069) -> (-22.5036, 14.6503)
  line L355 (-23.7189, 7.7582) -> (-23.2265, 7.6713)
  line L356 (-22.0112, 14.5634) -> (-22.5036, 14.6503)
  line L357 (-22.5032, 14.6526) -> (-23.7189, 7.7582)
  line L358 (-23.2265, 7.6713) -> (-22.0108, 14.5658)
  line L359 (-21.133, 14.4588) -> (-21.3821, 14.4806)
  line L360 (-21.992, 7.5088) -> (-21.4939, 7.4652)
  line L361 (-20.884, 14.437) -> (-21.3821, 14.4806)
  line L362 (-21.3819, 14.483) -> (-21.992, 7.5088)
  line L363 (-21.4939, 7.4652) -> (-20.8838, 14.4394)
  line L364 (-19.75, 3.9105) -> (-20.25, 3.9105)
  line L365 (-20.25, 3.9105) -> (-20.25, 10.9113)
  line L366 (-20.25, 10.9113) -> (-19.75, 10.9113)
  line L367 (-19.75, 10.9113) -> (-19.75, 3.9105)
  line L368 (-19.75, 3.9105) -> (-20.25, 10.9113) construction
  line L369 (-20.25, 3.9105) -> (-19.75, 10.9113) construction
  point P0 (0, 0)
  point P1 (-20, 7.4109)
  dimension "d41" = 40
  dimension "d40" = 26
  dimension "d45" = 360
  constraints: 738 end point, 145 point on line, 6 midpoint, 3 parallel, 2 coincident, 2 point on circle, 1 centre point, 1 horizontal, 1 perpendicular, 868 other
  measures "d40" diameter of A1
extrude "Extrusion5" cut sketch "Skizze7" against normal blind 0.5 contours L65 L67 L0 | L0 L67 L64 L66 L68 L65 | L63 L60 L62 L0 | L0 L62 L59 L61 L63 | L58 L55 L57 L0 | L0 L57 L54 L56 L58 | L53 L50 L52 L0 | L0 L52 L49 L51 L53 | L48 L45 L47 L0 | L0 L44 L46 L48 | L328 L325 L327 L0 | L0 L327 L324 L326 | L323 L320 L322 L0 | L0 L322 L319 L321 L323 | L318 L315 L317 L0 | L0 L317 L314 L316 L318 | L313 L310 L312 L0 | L0 L312 L309 L311 L313 | L308 L305 L0 | L0 L305 L307 L304 L306 L308 | L6 L8 L366 L7 L2 | L366 L8 L3 L7 | L3 L367 L364 L365 | L11 L13 L10 L12 L9 | L16 L18 L15 L17 L14 | L21 L23 L20 L22 L19 | L26 L28 L25 L27 L24 | L31 L33 L30 L32 L29 | L36 L38 L35 L37 L34 | L41 L43 L40 L42 L39 | L71 L73 L70 L72 L69 | L76 L78 L75 L77 L74 | L81 L83 L80 L82 L79 | L86 L88 L85 L87 L84 | L91 L93 L90 L92 L89 | L96 L98 L95 L97 L94 | L276 L278 L275 L277 L274 | L281 L283 L280 L282 L279 | L286 L288 L285 L287 L284 | L291 L293 L290 L292 L289 | L296 L298 L295 L297 L294 | L301 L303 L300 L302 L299 | L331 L333 L330 L332 L329 | L336 L338 L335 L337 L334 | L341 L343 L340 L342 L339 | L346 L348 L345 L347 L344 | L351 L353 L350 L352 L349 | L356 L358 L355 L357 L354 | L361 L363 L360 L362 L359
sketch "Skizze8" plane through (20, 0, 0) normal (1, 0, 0) x (0, 0, -1)
  line L0 (-36.8943, 6.554) -> (-25.9409, 6.554) construction
  line L1 (-25.9409, 6.554) -> (-25.9409, 2.0357) construction
  line L2 (-25.9409, 2.0357) -> (-36.8943, 2.0357) construction
  line L3 (-36.8943, 2.0357) -> (-36.8943, 6.554) construction
  spline S0 degree 2 poles (-34.5175, 4.1062) (-34.5175, 3.8538) (-34.6792, 3.4227) (-34.8266, 3.2639) knots 0 0 0 1 2 2 2
  spline S1 degree 2 poles (-34.8266, 3.2639) (-34.9741, 3.105) (-35.4138, 2.9207) (-35.686, 2.9207) knots 0 0 0 1 2 2 2
  spline S2 degree 2 poles (-35.686, 2.9207) (-35.9356, 2.9207) (-36.4235, 3.0313) (-36.6022, 3.1192) knots 0 0 0 1 2 2 2
  line L4 (-36.6022, 3.1192) -> (-36.6022, 3.6156)
  line L5 (-36.6022, 3.6156) -> (-36.5681, 3.6156)
  spline S3 degree 2 poles (-36.5681, 3.6156) (-36.5142, 3.5759) (-36.3129, 3.4737) (-36.1909, 3.4284) knots 0 0 0 1 2 2 2
  spline S4 degree 2 poles (-36.1909, 3.4284) (-36.0519, 3.3801) (-35.8222, 3.3263) (-35.6775, 3.3263) knots 0 0 0 1 2 2 2
  spline S5 degree 2 poles (-35.6775, 3.3263) (-35.5357, 3.3263) (-35.2691, 3.4284) (-35.1727, 3.539) knots 0 0 0 1 2 2 2
  spline S6 degree 2 poles (-35.1727, 3.539) (-35.0847, 3.6439) (-34.994, 3.9219) (-34.994, 4.1091) knots 0 0 0 1 2 2 2
  spline S7 degree 2 poles (-34.994, 4.1091) (-34.994, 4.2963) (-35.0961, 4.5345) (-35.1925, 4.6139) knots 0 0 0 1 2 2 2
  spline S8 degree 2 poles (-35.1925, 4.6139) (-35.2918, 4.7019) (-35.5868, 4.7756) (-35.7655, 4.7756) knots 0 0 0 1 2 2 2
  spline S9 degree 2 poles (-35.7655, 4.7756) (-35.9583, 4.7756) (-36.3412, 4.716) (-36.4575, 4.6905) knots 0 0 0 1 2 2 2
  line L6 (-36.4575, 4.6905) -> (-36.4575, 6.4944)
  line L7 (-36.4575, 6.4944) -> (-34.5373, 6.4944)
  line L8 (-34.5373, 6.4944) -> (-34.5373, 6.0831)
  line L9 (-34.5373, 6.0831) -> (-36.0065, 6.0831)
  line L10 (-36.0065, 6.0831) -> (-36.0065, 5.15)
  spline S10 degree 2 poles (-36.0065, 5.15) (-35.9215, 5.1613) (-35.7569, 5.1699) (-35.6889, 5.1699) knots 0 0 0 1 2 2 2
  spline S11 degree 2 poles (-35.6889, 5.1699) (-35.4194, 5.1699) (-35.0479, 5.0819) (-34.8777, 4.9515) knots 0 0 0 1 2 2 2
  spline S12 degree 2 poles (-34.8777, 4.9515) (-34.7047, 4.821) (-34.5175, 4.4239) (-34.5175, 4.1062) knots 0 0 0 1 2 2 2
  spline S13 degree 2 poles (-32.2399, 5.6605) (-32.2399, 5.2833) (-32.7561, 4.7671) (-33.1334, 4.7671) knots 0 0 0 1 2 2 2
  spline S14 degree 2 poles (-33.1334, 4.7671) (-33.5078, 4.7671) (-34.0296, 5.2805) (-34.0296, 5.6605) knots 0 0 0 1 2 2 2
  spline S15 degree 2 poles (-34.0296, 5.6605) (-34.0296, 6.0378) (-33.5134, 6.554) (-33.1334, 6.554) knots 0 0 0 1 2 2 2
  spline S16 degree 2 poles (-33.1334, 6.554) (-32.7561, 6.554) (-32.2399, 6.0378) (-32.2399, 5.6605) knots 0 0 0 1 2 2 2
  spline S17 degree 2 poles (-32.6086, 5.6605) (-32.6086, 5.8874) (-32.9093, 6.1966) (-33.1334, 6.1966) knots 0 0 0 1 2 2 2
  spline S18 degree 2 poles (-33.1334, 6.1966) (-33.3603, 6.1966) (-33.6609, 5.8874) (-33.6609, 5.6605) knots 0 0 0 1 2 2 2
  spline S19 degree 2 poles (-33.6609, 5.6605) (-33.6609, 5.4308) (-33.3546, 5.1245) (-33.1334, 5.1245) knots 0 0 0 1 2 2 2
  spline S20 degree 2 poles (-33.1334, 5.1245) (-32.9093, 5.1245) (-32.6086, 5.4365) (-32.6086, 5.6605) knots 0 0 0 1 2 2 2
  point P0 (0, 0)
  constraints: 2 other
extrude "Extrusion7" cut sketch "Skizze8" against normal blind 0.5
sketch "Skizze9" plane through (0, 0, 40) normal (0, 0, 1) x (1, 0, 0)
  line L0 (8.7628, 14.6502) -> (17.7993, 14.6502) construction
  line L1 (17.7993, 14.6502) -> (17.7993, 9.8581) construction
  line L2 (17.7993, 9.8581) -> (8.7628, 9.8581) construction
  line L3 (8.7628, 9.8581) -> (8.7628, 14.6502) construction
  line L4 (11.0006, 11.0793) -> (9.2931, 11.0793)
  line L5 (9.2931, 11.0793) -> (9.2931, 11.4367)
  line L6 (9.2931, 11.4367) -> (9.9285, 11.4367)
  line L7 (9.9285, 11.4367) -> (9.9285, 13.7823)
  line L8 (9.9285, 13.7823) -> (9.2931, 13.7823)
  line L9 (9.2931, 13.7823) -> (9.2931, 14.1028)
  spline S0 degree 2 poles (9.2931, 14.1028) (9.6534, 14.1028) (9.9937, 14.307) (10.0164, 14.5907) knots 0 0 0 1 2 2 2
  line L10 (10.0164, 14.5907) -> (10.3794, 14.5907)
  line L11 (10.3794, 14.5907) -> (10.3794, 11.4367)
  line L12 (10.3794, 11.4367) -> (11.0006, 11.4367)
  line L13 (11.0006, 11.4367) -> (11.0006, 11.0793)
  spline S1 degree 2 poles (13.8227, 12.8293) (13.8227, 11.8877) (13.2753, 11.0056) (12.7052, 11.0056) knots 0 0 0 1 2 2 2
  spline S2 degree 2 poles (12.7052, 11.0056) (12.1266, 11.0056) (11.5849, 11.9047) (11.5849, 12.8265) knots 0 0 0 1 2 2 2
  spline S3 degree 2 poles (11.5849, 12.8265) (11.5849, 13.7738) (12.1323, 14.6502) (12.7052, 14.6502) knots 0 0 0 1 2 2 2
  spline S4 degree 2 poles (12.7052, 14.6502) (13.281, 14.6502) (13.8227, 13.7426) (13.8227, 12.8293) knots 0 0 0 1 2 2 2
  spline S5 degree 2 poles (13.2214, 11.7629) (13.2895, 11.9359) (13.3462, 12.4691) (13.3462, 12.8293) knots 0 0 0 1 2 2 2
  spline S6 degree 2 poles (13.3462, 12.8293) (13.3462, 13.1895) (13.2895, 13.7199) (13.2186, 13.8986) knots 0 0 0 1 2 2 2
  spline S7 degree 2 poles (13.2186, 13.8986) (13.1477, 14.0773) (12.9009, 14.2617) (12.7052, 14.2617) knots 0 0 0 1 2 2 2
  spline S8 degree 2 poles (12.7052, 14.2617) (12.5095, 14.2617) (12.2571, 14.0773) (12.1833, 13.8929) knots 0 0 0 1 2 2 2
  spline S9 degree 2 poles (12.1833, 13.8929) (12.1124, 13.7142) (12.0614, 13.1697) (12.0614, 12.8265) knots 0 0 0 1 2 2 2
  spline S10 degree 2 poles (12.0614, 12.8265) (12.0614, 12.4578) (12.1068, 11.9642) (12.1805, 11.7714) knots 0 0 0 1 2 2 2
  spline S11 degree 2 poles (12.1805, 11.7714) (12.2486, 11.5899) (12.501, 11.3941) (12.7052, 11.3941) knots 0 0 0 1 2 2 2
  spline S12 degree 2 poles (12.7052, 11.3941) (12.8981, 11.3941) (13.1505, 11.5785) (13.2214, 11.7629) knots 0 0 0 1 2 2 2
  spline S13 degree 2 poles (16.0435, 13.7454) (16.0435, 13.3682) (15.5273, 12.852) (15.1501, 12.852) knots 0 0 0 1 2 2 2
  spline S14 degree 2 poles (15.1501, 12.852) (14.7757, 12.852) (14.2538, 13.3654) (14.2538, 13.7454) knots 0 0 0 1 2 2 2
  spline S15 degree 2 poles (14.2538, 13.7454) (14.2538, 14.1227) (14.77, 14.6389) (15.1501, 14.6389) knots 0 0 0 1 2 2 2
  spline S16 degree 2 poles (15.1501, 14.6389) (15.5273, 14.6389) (16.0435, 14.1227) (16.0435, 13.7454) knots 0 0 0 1 2 2 2
  spline S17 degree 2 poles (15.6748, 13.7454) (15.6748, 13.9723) (15.3742, 14.2815) (15.1501, 14.2815) knots 0 0 0 1 2 2 2
  spline S18 degree 2 poles (15.1501, 14.2815) (14.9232, 14.2815) (14.6226, 13.9723) (14.6226, 13.7454) knots 0 0 0 1 2 2 2
  spline S19 degree 2 poles (14.6226, 13.7454) (14.6226, 13.5157) (14.9289, 13.2094) (15.1501, 13.2094) knots 0 0 0 1 2 2 2
  spline S20 degree 2 poles (15.1501, 13.2094) (15.3742, 13.2094) (15.6748, 13.5214) (15.6748, 13.7454) knots 0 0 0 1 2 2 2
  point P0 (0, 0)
  constraints: 2 other
extrude "Extrusion8" cut sketch "Skizze9" against normal blind 0.5
